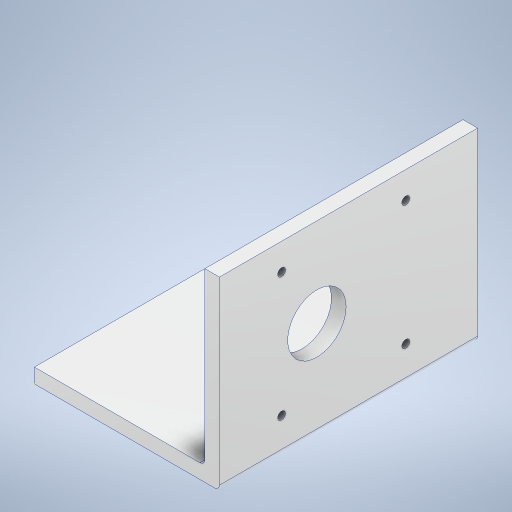
# Autodesk Inventor part: MOTOR BRACKET
Saved by Autodesk Inventor 2023 (Build 270158000, 158)
## iProperties
Created: 2022-09-15
Part Number: MOTOR BRACKET
Material: Aluminum 6061
Document SubType Name: Modeling
Designer: D.C. Eksteen
Density: 2.7 g/cm^3
Appearance: Aluminum - Flat
Author: D.C. Eksteen
Autodesk Inventor part; units mm, degrees
ref_plane "YZ Plane" through (0, 0, 0) normal (1, 0, 0) x (0, 1, 0)
ref_plane "XZ Plane" through (0, 0, 0) normal (0, 1, 0) x (-1, 0, 0)
ref_plane "XY Plane" through (0, 0, 0) normal (0, 0, 1) x (1, 0, 0)
sketch "Sketch1" plane through (0, 0, 0) normal (0, 0, 1) x (1, 0, 0)
  point P0 (0, 0)
sketch "Sketch2" plane through (0, 0, 0) normal (0, 0, 1) x (1, 0, 0)
  line L0 (0, 0) -> (76, 0)
  line L1 (76, 0) -> (76, 76)
  line L2 (76, 76) -> (0, 76)
  line L3 (0, 76) -> (0, 0)
  line L4 (70, 6) -> (6, 6)
  line L5 (6, 6) -> (6, 70)
  line L6 (6, 70) -> (70, 70)
  line L7 (70, 70) -> (70, 6)
  line L8 (6, 6) -> (0, 6)
  line L9 (70, 70) -> (70, 76)
  dimension "d0" = 76
  dimension "d1" = 76
  dimension "d2" = 6
  constraints: 20 end point, 4 parallel, 4 perpendicular, 2 point on line, 1 horizontal, 3 other
  measures "d0" distance of L2.end L1.end
  measures "d1" distance of L1.end L0.end
  measures "d2" distance between parallel lines of L0 L4
extrude "Extrusion1" add sketch "Sketch2" against normal blind 106 contours L3 L8 L4 L7 L9 L2 L1 L0
fillet "Fillet1" radius 2 2 edges at (76, 0, -53) (70, 6, -53)
sketch "Sketch3" plane through (76, 76, 0) normal (1, 0, 0) x (0, 0, -1)
  line L0 (0, -76) -> (106, -76) projected
  line L1 (106, -74) -> (0, -74) projected
  line L2 (106, 0) -> (106, -74) projected
  line L3 (0, 0) -> (106, 0) projected
  line L4 (0, -74) -> (0, 0) projected
  circle A0 centre (40, -36.5) radius 12
  dimension "d6" = 24
  dimension "d7" = 40
  dimension "d8" = 39.5
  constraints: 1 centre point
  measures "d6" diameter of A0
  measures "d7" distance from line of L4 A0.centre
  measures "d8" distance from line of L0 A0.centre
extrude "Extrusion2" cut sketch "Sketch3" against normal blind 76 contours A0
sketch "Sketch4" plane through (70, 76, -106) normal (-1, 0, 0) x (0, 0, 1)
  line L0 (25, -6.5) -> (85, -6.5)
  line L1 (85, -6.5) -> (85, -66.5)
  line L2 (85, -66.5) -> (25, -66.5)
  line L3 (25, -66.5) -> (25, -6.5)
  circle A0 centre (66, -36.5) radius 12 projected
  circle A1 centre (66, -36.5) radius 12 projected
  line L4 (106, -68) -> (0, -68) projected
  line L5 (106, 0) -> (106, -68) projected
  line L6 (106, 0) -> (0, 0) projected
  line L7 (0, -68) -> (0, 0) projected
  line L8 (80.5, -11) -> (29.5, -11) construction
  line L9 (29.5, -11) -> (29.5, -62) construction
  line L10 (29.5, -62) -> (80.5, -62) construction
  line L11 (80.5, -62) -> (80.5, -11) construction
  point P0 (106, -76)
  dimension "d11" = 19
  dimension "d12" = 60
  dimension "d13" = 60
  dimension "d14" = 30
  dimension "d15" = 4.5
  constraints: 16 end point, 4 coincident, 4 parallel, 2 perpendicular, 1 horizontal, 3 other
  measures "d11" distance from line of A0.centre L1
  measures "d12" distance between parallel lines of L3 L1
  measures "d13" distance between parallel lines of L2 L0
  measures "d14" distance from line of A0.centre L2
  measures "d15" distance between parallel lines of L0 L8
hole "Hole1" at (70, 65, -76.5) at (70, 65, -25.5) at (70, 14, -25.5) at (70, 14, -76.5) direction (1, 0, 0) diameter 3.242 end through all thread size "M4x0.7" class "6H" standard "ANSI Metric M Profile"
body "Solid1"
